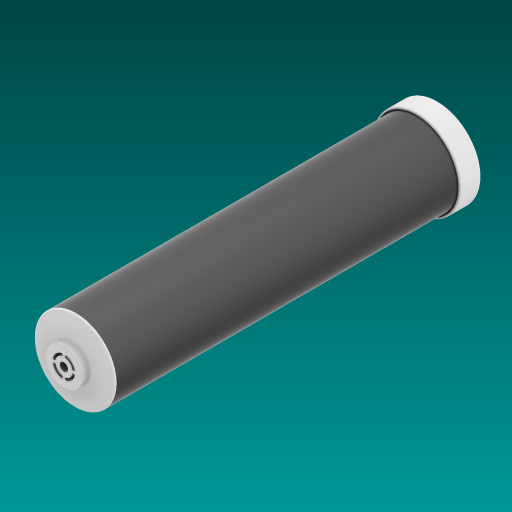
# Autodesk Inventor part: 2.5X12inAirTank
Saved by Autodesk Inventor 2024.2 (Build 282272000, 272)
## iProperties
Created: 2024-02-17
Part Number: 2.5X12inAirTank
Material: Generic
Document SubType Name: Modeling
Designer: colli
Density: 1 g/cm^3
Appearance: Cool White
Author: colli
Autodesk Inventor part; units mm, degrees
ref_plane "YZ Plane" through (0, 0, 0) normal (1, 0, 0) x (0, 1, 0)
ref_plane "XZ Plane" through (0, 0, 0) normal (0, 1, 0) x (-1, 0, 0)
ref_plane "XY Plane" through (0, 0, 0) normal (0, 0, 1) x (1, 0, 0)
sketch "Sketch1" plane through (0, 0, 0) normal (0, 0, 1) x (1, 0, 0)
  circle A0 centre (0, 0) radius 14.605
  dimension "d0" = 29.21
  constraints: 1 centre point, 1 coincident
  measures "d0" diameter of A0
extrude "Extrusion1" add sketch "Sketch1" along normal blind 306.705
sketch "Sketch3" plane through (0, 0, 0) normal (0, 0, -1) x (-1, 0, 0)
  circle A0 centre (0, 0) radius 34.925
  circle A1 centre (0, 0) radius 14.605
  dimension "d4" = 69.85
  constraints: 2 centre point, 2 coincident
  measures "d4" diameter of A0
extrude "Extrusion2" add sketch "Sketch3" against normal blind 25.4 contours A0 | A1
extrude "Extrusion3" cut sketch "Sketch3" against normal blind 8.382
sketch "Sketch4" plane through (0, 0, 25.4) normal (0, 0, 1) x (1, 0, 0)
  circle A0 centre (0, 0) radius 32.385
  dimension "d9" = 64.77
  constraints: 1 centre point, 1 coincident
  measures "d9" diameter of A0
extrude "Extrusion4" add sketch "Sketch4" along normal blind 272.923
fillet "Fillet1" radius 1.27 3 edges at (34.925, 0, 25.4) (34.925, 0, 8.382) (-32.385, 0, 298.323)
sketch "Sketch5" plane through (0, 0, 0) normal (1, 0, 0) x (0, 1, 0)
  line L0 (-14.605, 0) -> (14.605, 0) projected
  line L1 (14.605, 0) -> (14.605, 6.35)
  line L2 (14.605, 8.382) -> (14.605, 0) projected
  line L3 (33.655, 8.382) -> (-33.655, 8.382) projected
  line L4 (14.605, 6.35) -> (33.655, 8.382)
  line L5 (0, -61.341) -> (0, 368.046) projected
  point P0 (0, 0)
  dimension "d13" = 6.35
  constraints: 4 end point, 1 point on line
  measures "d13" distance of L0.end L1.end
revolve "Revolution1" add sketch "Sketch5" angle 360 about axis through (0, 0, -10) along (0, 0, 1) contours L2 L3 L4
sketch "Sketch6" plane through (0, 0, 0) normal (0, 1, 0) x (-1, 0, 0)
  line L0 (14.605, 306.705) -> (-14.605, 306.705) projected
  line L1 (14.605, 306.705) -> (14.605, 300.355)
  line L2 (14.605, 298.323) -> (14.605, 306.705) projected
  line L3 (14.605, 300.355) -> (31.115, 298.323)
  arc A0 (32.385, 297.053) -> (31.115, 298.323) centre (31.115, 297.053) ccw projected
  line L4 (14.605, 298.323) -> (-14.605, 298.323) projected
  line L5 (14.605, 306.705) -> (-14.605, 306.705) projected
  line L6 (-31.115, 298.323) -> (31.115, 298.323) projected
  line L7 (0, -61.341) -> (0, 368.046) projected
  point P0 (0, 0)
  dimension "d15" = 6.35
  constraints: 4 end point, 1 point on circle, 1 point on line
  measures "d15" distance of L0.start L1.end
revolve "Revolution2" add sketch "Sketch6" angle 360 about axis through (0, 0, -10) along (0, 0, 1) contours L3 L6 L2
sketch "Sketch7" plane through (0, 0, 0) normal (0, 0, -1) x (-1, 0, 0)
  circle A0 centre (0, 0) radius 14.605 projected
  circle A1 centre (0, 0) radius 3.175
  circle A2 centre (0, 0) radius 9.525
  line L0 (3.175, 0) -> (9.525, 0)
  line L1 (0, -3.175) -> (0, -9.525)
  line L2 (9.525, 0) -> (7.62, 0)
  line L3 (0, -9.525) -> (0, -7.62)
  line L4 (0, -7.62) -> (1.905, -7.62)
  line L5 (1.905, -7.62) -> (1.905, -5.715)
  line L6 (7.62, 0) -> (7.62, -1.905)
  line L7 (7.62, -1.905) -> (5.715, -1.905)
  arc A3 (1.905, -7.62) -> (7.62, -1.905) centre (0, 0) ccw construction
  arc A4 (2.136, -8.5441) -> (8.5441, -2.136) centre (0, 0) ccw
  arc A5 (1.674, -6.6959) -> (6.6959, -1.674) centre (0, 0) ccw
  arc A6 (1.674, -6.6959) -> (2.136, -8.5441) centre (1.905, -7.62) ccw
  arc A7 (8.5441, -2.136) -> (6.6959, -1.674) centre (7.62, -1.905) ccw
  dimension "d17" = 6.35
  dimension "d18" = 19.05
  dimension "d19" = 1.905
  dimension "d20" = 1.905
  dimension "d21" = 1.905
  dimension "d22" = 1.905
  dimension "d23" = 1.905
  constraints: 16 end point, 14 point on circle, 7 centre point, 4 tangent, 3 coincident, 2 horizontal, 2 perpendicular, 2 point on line, 2 vertical
  measures "d17" diameter of A1
  measures "d18" diameter of A2
  measures "d19" distance of L0.end L2.end
  measures "d20" distance of L1.end L3.end
  measures "d21" distance of L3.end L4.end
  measures "d22" distance of L2.end L6.end
  measures "d23" diameter of A6
extrude "Extrusion5" cut sketch "Sketch7" against normal blind 6.35 contours A7 A4 A6 L4 L5 A5 L7 L6 | L6 L7 A5 A7 | A6 A5 L5 L4
pattern_circular "Circular Pattern1" count 4 over 360 about axis through (0, 0, -10) along (0, 0, 1) of "Extrusion5"
sketch "Sketch8" plane through (0, 0, 0) normal (0, 0, -1) x (-1, 0, 0)
  circle A0 centre (0, 0) radius 6.35
  dimension "d29" = 12.7
  constraints: 1 centre point, 1 coincident
  measures "d29" diameter of A0
sketch "Sketch9" plane through (0, 0, 25.4) normal (0, 0, 1) x (1, 0, 0)
  circle A0 centre (0, 0) radius 3.2385
  circle A1 centre (0, 0) radius 31.75
  dimension "d30" = 6.477
  dimension "d31" = 63.5
  constraints: 2 centre point, 2 coincident
  measures "d30" diameter of A0
  measures "d31" diameter of A1
extrude "Extrusion6" cut sketch "Sketch9" along normal blind 271.653 contours A0 | A1
sketch "Sketch10" plane through (0, 0, 0) normal (0, 0, -1) x (-1, 0, 0)
  circle A0 centre (0, 0) radius 3.175
  dimension "d34" = 6.35
  constraints: 1 centre point, 1 coincident
  measures "d34" diameter of A0
extrude "Extrusion7" cut sketch "Sketch10" along normal through all both and the other way through all
extrude "Extrusion8" cut sketch "Sketch9" against normal blind 15.24 contours A0 | A1
sketch "Sketch11" plane through (0, 0, 306.705) normal (0, 0, 1) x (1, 0, 0)
  circle A0 centre (0, 0) radius 14.605
  circle A1 centre (0, 0) radius 3.175
  circle A2 centre (0, 0) radius 9.525
  line L0 (3.175, 0) -> (9.525, 0)
  line L1 (0, -3.175) -> (0, -9.525)
  line L2 (9.525, 0) -> (7.62, 0)
  line L3 (0, -9.525) -> (0, -7.62)
  line L4 (0, -7.62) -> (1.905, -7.62)
  line L5 (1.905, -7.62) -> (1.905, -5.9372)
  line L6 (7.62, 0) -> (7.62, -1.905)
  line L7 (7.62, -1.905) -> (5.3447, -1.905)
  arc A3 (1.905, -7.62) -> (7.62, -1.905) centre (0, 0) ccw construction
  arc A4 (2.136, -8.5441) -> (8.5441, -2.136) centre (0, 0) ccw
  arc A5 (1.674, -6.6959) -> (6.6959, -1.674) centre (0, 0) ccw
  arc A6 (1.674, -6.6959) -> (2.136, -8.5441) centre (1.905, -7.62) ccw
  arc A7 (8.5441, -2.136) -> (6.6959, -1.674) centre (7.62, -1.905) ccw
  dimension "d39" = 6.35
  dimension "d40" = 19.05
  dimension "d41" = 1.905
  dimension "d42" = 1.905
  dimension "d43" = 1.905
  dimension "d44" = 1.905
  dimension "d45" = 1.905
  constraints: 16 end point, 14 point on circle, 8 centre point, 5 coincident, 4 tangent, 2 horizontal, 2 perpendicular, 2 point on line, 2 vertical
  measures "d39" diameter of A1
  measures "d40" diameter of A2
  measures "d41" distance of L0.end L2.end
  measures "d42" distance of L1.end L3.end
  measures "d43" distance of L3.end L4.end
  measures "d44" distance of L2.end L6.end
  measures "d45" diameter of A6
extrude "Extrusion9" cut sketch "Sketch11" against normal blind 6.35 contours A7 A4 A6 L4 L5 A5 L7 L6 | L6 L7 A5 A7 | A6 A5 L5 L4
pattern_circular "Circular Pattern2" count 4 over 360 about axis through (0, 0, -10) along (0, 0, 1) of "Extrusion9"
body "Solid1"
